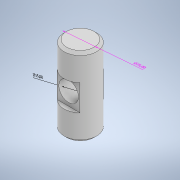
# Autodesk Inventor part: Pino Plataforma Deslizante
Saved by Autodesk Inventor 2021 (Build 250183000, 183)
## iProperties
Created: 2021-08-18
Part Number: Pino Plataforma Deslizante
Material: Generic
Document SubType Name: Modeling
Designer: guilh
Density: 1 g/cm^3
Appearance: Default
Author: guilh
Autodesk Inventor part; units mm, degrees
ref_plane "YZ Plane" through (0, 0, 0) normal (1, 0, 0) x (0, 1, 0)
ref_plane "XZ Plane" through (0, 0, 0) normal (0, 1, 0) x (-1, 0, 0)
ref_plane "XY Plane" through (0, 0, 0) normal (0, 0, 1) x (1, 0, 0)
sketch "Sketch1" plane through (0, 0, 0) normal (0, 1, 0) x (-1, 0, 0)
  circle A0 centre (0, 0) radius 12.5
  dimension "d0" = 25
  constraints: 1 centre point, 1 coincident
  measures "d0" diameter of A0
extrude "Extrusion1" add sketch "Sketch1" along normal blind 60
sketch "Sketch2" plane through (0, 0, 0) normal (0, 0, 1) x (1, 0, 0)
  line L0 (0, 0) -> (0, 30)
  circle A0 centre (0, 30) radius 7.5
  dimension "d3" = 30
  dimension "d4" = 15
  constraints: 2 end point, 1 centre point, 1 coincident, 1 vertical
  measures "d3" distance of L0.start L0.end
  measures "d4" diameter of A0
extrude "Extrusion2" cut sketch "Sketch2" along normal mid plane 60
chamfer "Chamfer1" distance 2 angle 45 2 edges at (12.5, 60, 0) (12.5, 0, 0)
sketch "Sketch3" plane through (0, 0, 0) normal (1, 0, 0) x (0, 1, 0)
  line L0 (0, 0) -> (20, 0)
  line L1 (20, 0) -> (20, -9)
  line L2 (2, -12.5) -> (58, -12.5) projected
  line L3 (20, -9) -> (40, -9)
  line L4 (40, -9) -> (40, 9)
  line L5 (40, 9) -> (20, 9)
  line L6 (20, 9) -> (20, 0)
  line L7 (40, -9) -> (40, -15.8527)
  line L8 (40, -15.8527) -> (20, -15.8527)
  line L9 (20, -15.8527) -> (20, -9)
  line L10 (20, 9) -> (20, 19.7516)
  line L11 (20, 19.7516) -> (40, 19.7516)
  line L12 (40, 19.7516) -> (40, 9)
  dimension "d20" = 20
  dimension "d21" = 9
  dimension "d22" = 20
  dimension "d23" = 18
  constraints: 24 end point, 7 perpendicular, 3 point on line, 2 collinear, 1 horizontal, 1 vertical
  measures "d20" distance of L0.start L0.end
  measures "d21" distance of L0.end L1.end
  measures "d22" distance of L1.end L3.end
  measures "d23" distance of L3.end L4.end
extrude "Extrusion3" cut sketch "Sketch3" along normal mid plane 25 contours L3 L7 L2 L9 | L10 L11 L12 L5 | L2 L7 L8 L9
body "Solid1"
